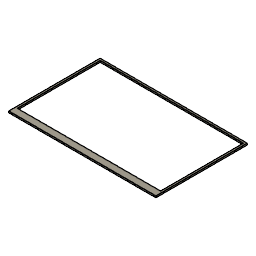
PokrywaGóra (Autodesk Fusion 360 design; units mm, degrees)
part number: 2025-11-11-11-18-34-591
Autodesk Fusion 360 part; units mm, degrees
sketch "Szkic1" plane through (0, 0, 0) normal (0, 0, 1) x (1, 0, 0)
  line L0 (-50, 50) -> (320, 50)
  line L1 (320, 50) -> (320, -179.9)
  line L2 (320, -179.9) -> (-50, -179.9)
  line L3 (-50, -179.9) -> (-50, 50)
  line L4 (-45, 45) -> (315, 45)
  line L5 (315, 45) -> (315, -163)
  line L6 (315, -163) -> (-45, -163)
  line L7 (-45, -163) -> (-45, 45)
  dimension "d1" = 370
  dimension "d2" = 229.9
  dimension "d3" = 360
  dimension "d4" = 208
  dimension "d6" = 5
  dimension "d7" = 5
  constraint horizontal L0
  constraint vertical L1
  constraint horizontal L2
  constraint vertical L3
  constraint horizontal L4
  constraint vertical L5
  constraint horizontal L6
  constraint vertical L7
  measures "d1" distance of L0.start L0.end
  measures "d2" distance of L0.start L2.end
  measures "d3" distance of L4.start L4.end
  measures "d4" distance of L4.start L6.end
  measures "d6" distance of L0 L4
  measures "d7" distance of L3 L7
extrude "Wyciągnięcie proste1" add sketch "Szkic1" along normal blind 4
